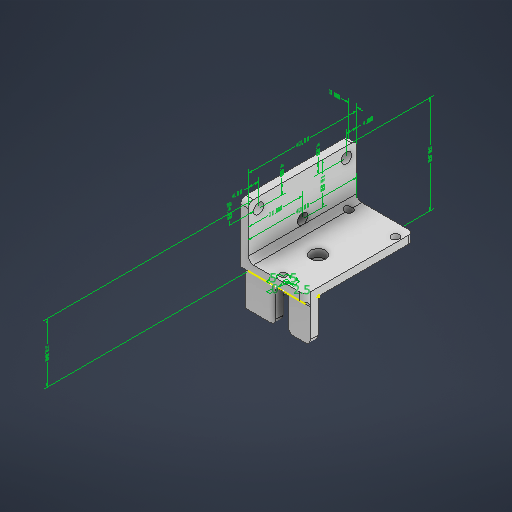
# Autodesk Inventor part: MotorBracket
Saved by Autodesk Inventor 2026 (Build 300175000, 175)
## iProperties
Created: 2025-07-22
Part Number: MotorBracket
Material: Generic
Document SubType Name: Modeling
Designer: jsmal
Density: 1 g/cm^3
Appearance: Default
Author: jsmal
Autodesk Inventor part; units mm, degrees
ref_plane "YZ Plane" through (0, 0, 0) normal (1, 0, 0) x (0, 1, 0)
ref_plane "XZ Plane" through (0, 0, 0) normal (0, 1, 0) x (-1, 0, 0)
ref_plane "XY Plane" through (0, 0, 0) normal (0, 0, 1) x (1, 0, 0)
sketch "Sketch1" plane through (0, 0, 0) normal (0, 1, 0) x (-1, 0, 0)
  line L0 (0, 0) -> (22, 0)
  line L1 (22, 0) -> (22, -37)
  line L2 (22, -37) -> (0, -37)
  line L3 (0, -37) -> (0, 0)
  dimension "d0" = 22
  dimension "d1" = 37
  constraints: 8 end point, 2 parallel, 1 horizontal, 1 perpendicular
  measures "d0" distance of L1.end L2.end
  measures "d1" distance of L0.end L1.end
extrude "Extrusion1" add sketch "Sketch1" along normal blind 3
sketch "Sketch2" plane through (0, 3, 0) normal (0, 1, 0) x (1, 0, 0)
  line L0 (0, 0) -> (0, 37) projected
  line L1 (-22, 0) -> (0, 0) projected
  point P0 (-11, 11)
  dimension "d4" = 11
  dimension "d12" = 11
  measures "d4" distance from line of L0 point (-11, 11)
  measures "d12" distance from line of L1 point (-11, 11)
hole "Hole1" at (-11, 3, -11) direction (0, -1, 0) diameter 5.8 depth 3 tip angle 118
sketch "Sketch3" plane through (0, 3, 0) normal (0, 1, 0) x (1, 0, 0)
  line L0 (0, 37) -> (-22, 37) projected
  line L1 (0, 0) -> (0, 37) projected
  line L2 (-22, 37) -> (-22, 0) projected
  point P0 (-20, 32)
  point P1 (-2, 32)
  dimension "d13" = 5
  dimension "d21" = 5
  dimension "d22" = 2
  dimension "d23" = 2
  measures "d13" distance from line of L0 point (-20, 32)
  measures "d21" distance from line of L0 point (-2, 32)
  measures "d22" distance from line of L1 point (-2, 32)
  measures "d23" distance from line of L2 point (-20, 32)
hole "Hole2" at (-20, 3, -32) at (-2, 3, -32) direction (0, -1, 0) diameter 3 depth 3 tip angle 118
sketch "Sketch4" plane through (-22, 0, 0) normal (0, 0, 1) x (1, 0, 0)
  line L0 (22, 0) -> (0, 0) projected
  line L1 (22, 3) -> (0, 3) projected
  line L2 (0, 0) -> (22, 0)
  line L3 (22, 0) -> (22, 3)
  line L4 (22, 3) -> (0, 3)
  line L5 (0, 3) -> (0, 0)
  constraints: 8 end point, 2 parallel, 1 horizontal, 1 perpendicular
extrude "Extrusion2" add sketch "Sketch4" along normal blind 5
sketch "Sketch5" plane through (0, 3, 0) normal (0, 1, 0) x (1, 0, 0)
  line L0 (0, 37) -> (0, -5) projected
  line L1 (0, -5) -> (-22, -5) projected
  point P0 (0, 0)
  point P1 (-11, -2.5)
  dimension "d26" = 11
  dimension "d27" = 2.5
  measures "d26" distance from line of L0 point (-11, -2.5)
  measures "d27" distance from line of L1 point (-11, -2.5)
hole "Hole3" at (-11, 3, 2.5) direction (0, -1, 0) diameter 2.5 depth 3 tip angle 118
sketch "Sketch6" plane through (-22, 0, -37) normal (-1, 0, 0) x (0, 0, 1)
  line L0 (0, 3) -> (42, 3) projected
  line L1 (0, 0) -> (42, 0)
  line L2 (42, 0) -> (42, 3)
  line L3 (42, 3) -> (0, 3)
  line L4 (0, 3) -> (0, 0)
  point P0 (37, 0)
  point P1 (0, 3)
  constraints: 8 end point, 2 parallel, 1 horizontal, 1 perpendicular
extrude "Extrusion3" add sketch "Sketch6" along normal blind 3
sketch "Sketch7" plane through (0, 3, 0) normal (0, 1, 0) x (1, 0, 0)
  line L0 (0, -5) -> (-25, -5) projected
  line L1 (0, 37) -> (-25, 37) projected
  line L2 (-25, -5) -> (-22, -5)
  line L3 (-22, -5) -> (-22, 37)
  line L4 (-22, 37) -> (-25, 37)
  line L5 (-25, 37) -> (-25, -5)
  point P0 (0, 0)
  dimension "d37" = 3
  constraints: 8 end point, 2 parallel, 1 horizontal, 1 perpendicular, 1 point on line
  measures "d37" distance of L4.end L3.end
extrude "Extrusion4" add sketch "Sketch7" along normal blind 20 and the other way blind 18
sketch "Sketch9" plane through (0, 0, 0) normal (0, -1, 0) x (1, 0, 0)
  line L0 (-8.5, 5) -> (-13.5, 5)
  line L1 (-13.5, 5) -> (-13.5, 0)
  line L2 (-13.5, 0) -> (-8.5, 0)
  line L3 (-8.5, 0) -> (-8.5, 5)
  line L4 (0, 5) -> (-22, 5) projected
  circle A0 centre (-11, 2.5) radius 1.25 projected
  point P0 (0, 0)
  point P1 (-11, 5)
  dimension "d44" = 5
  dimension "d45" = 5
  dimension "d46" = 0
  dimension "d47" = 2.5
  constraints: 8 end point, 2 parallel, 1 horizontal, 1 midpoint, 1 perpendicular
  measures "d44" distance of L2.end L1.end
  measures "d45" distance of L1.end L0.end
  measures "d46" distance from line of L4 point (-11, 5)
  measures "d47" distance from line of L3 A0.centre
sketch "Sketch10" plane through (0, 0, 0) normal (0, -1, 0) x (1, 0, 0)
  line L0 (0, -37) -> (0, 5) projected
  line L1 (-8.5001, 0) -> (0, 0)
  line L2 (0, 0) -> (0, 3)
  line L3 (0, 3) -> (-8.5001, 3)
  line L4 (-8.5001, 3) -> (-8.5001, 0)
  line L5 (-22, 5) -> (-22, -37) projected
  line L6 (-13.5, 0) -> (-22, 0)
  line L7 (-22, 0) -> (-22, 3)
  line L8 (-22, 3) -> (-13.5, 3)
  line L9 (-13.5, 3) -> (-13.5, 0)
  point P0 (0, 0)
  point P1 (0, 0)
  dimension "d48" = 3
  dimension "d49" = 3
  constraints: 16 end point, 4 parallel, 2 horizontal, 2 perpendicular, 2 point on line
  measures "d48" distance of L2.end L1.end
  measures "d49" distance of L6.end L7.end
extrude "Extrusion6" add sketch "Sketch10" along normal blind 15
sketch "Sketch11" plane through (-22, -15, 5) normal (1, 0, 0) x (0, 0, -1)
  line L0 (2, 15) -> (0, 15) projected
  line L1 (2, 0) -> (5, 0) projected
  line L2 (0, 15) -> (2, 15)
  line L3 (2, 15) -> (2, 0)
  line L4 (2, 0) -> (0, 0)
  line L5 (0, 0) -> (0, 15)
  point P0 (5, 15)
  constraints: 8 end point, 2 parallel, 1 horizontal, 1 perpendicular
extrude "Extrusion7" cut sketch "Sketch11" against normal blind 15
sketch "Sketch12" plane through (-22, 3, 5) normal (1, 0, 0) x (0, 0, -1)
  line L0 (0, 20) -> (42, 20) projected
  line L1 (0, 0) -> (0, 20) projected
  line L2 (42, 0) -> (42, 20) projected
  line L3 (42, 0) -> (0, 0) projected
  point P0 (5, -3)
  point P1 (4, 16)
  point P2 (38, 16)
  point P3 (21, 4)
  dimension "d57" = 4
  dimension "d58" = 4
  dimension "d59" = 4
  dimension "d60" = 4
  dimension "d61" = 4
  dimension "d62" = 21
  measures "d57" distance from line of L0 point (4, 16)
  measures "d58" distance from line of L1 point (4, 16)
  measures "d59" distance from line of L0 point (38, 16)
  measures "d60" distance from line of L2 point (38, 16)
  measures "d61" distance from line of L3 point (21, 4)
  measures "d62" distance from line of L2 point (21, 4)
hole "Hole4" at (-22, 19, 1) at (-22, 19, -33) at (-22, 7, -16) direction (-1, 0, 0) diameter 4 depth 3 tip angle 118
fillet "Fillet1" radius 2 1 edges at (-22, 3, -16)
fillet "Fillet2" radius 2 8 edges at (-4.2501, 0, 3) (-19.25, 0, 3) (-13.5, -15, 1.5) (-8.5001, -15, 1.5) (-23.5, 23, -37) (-23.5, 23, 5) (0, 1.5, -37) (0, 1.5, 5)
fillet "Fillet3" radius 2 1 edges at (0, -15, 1.5)
body "Solid1"
